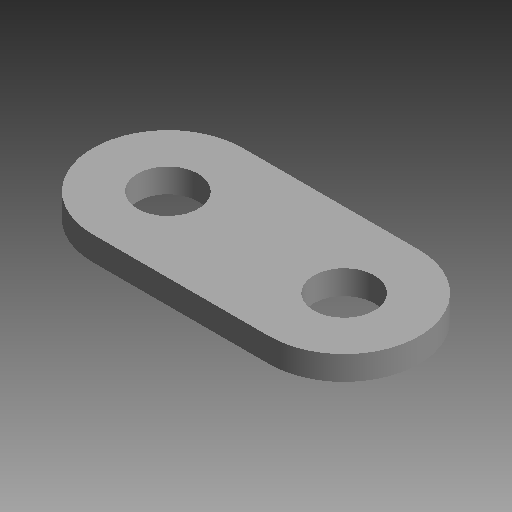
# Autodesk Inventor part: 06B - 1 RP- Link Plate
Saved by Autodesk Inventor 2019 (Build 230136000, 136)
## iProperties
Category: PARTsolutions
Company: KANA
Part Number: 06B - 1 RP- Link Plate
Material: 一般
Catalog Web Link: www.cadenas.de
Description: Standard Chain_Body1a-
Vendor: KANA
Document SubType Name: Modeling
Designer: partserver
Manufacturer: KANA
Mass: 0.145318 g
Surface Area: 3.08204 cm^2
Volume: 0.145318 cm^3
Density: 1 g/cm^3
Appearance: PSOLRGB-192-192-192
PSOL_IDENT_0: {$CADENAS_DATA\23d-libs\kana\roller_chain\standard_chain\standard_chain_body1_a.prj},194 {VTYP=3D},{
PSOL_IDENT_1: NB=06B - 1 RP- Link Plate},{LINA=06B - 1 RP},{NN=Standard Chain_Body1a},{DATE=04.07.2018 01:10:23},{
PSOL_IDENT_2: GEOMDATE=05.10.2016 10:14:00},{VERSION=},{LINEID=250},{WBVAR=NOL},{WBNUMERIC=NOL}  {NB=06B - 1 RP- L
PSOL_IDENT_3: ink Plate},{LINA=06B - 1 RP},{KT=DUMMY},{CNO=06B},{PT=RP},{NOL=1},{NOLX=1},{P=9.525},{R=6.350},{W=5.
PSOL_IDENT_4: 720},{T=1.300},{H=8.100},{D=3.280},{L=13.6},{C=10.24},{H2=8.100}
NB: 06B - 1 RP- Link Plate
NN: Standard Chain_Body1a
NBSYN: $CNO. - $NOL. $PT.- Link Plate
LINA: 06B - 1 RP
CATALOG: KANA
CNO: 06B
PT: RP
NOL: 1
P: 9.525
R: 6.35
W: 5.72
T: 1.3
H: 8.1
D: 3.28
H2: 8.1
SUPPLIER: KANA
ARTICLENO: 06B - 1 RP- Link Plate
BOMINFO: 06B - 1 RP
CREATOR: CADENAS GmbH
Title: 06B - 1 RP
Author: Cadenas PARTsolutions
Autodesk Inventor part; units mm, degrees
sketch "Sketch_4" plane through (0, 0, 0) normal (0, 0, 1) x (1, 0, 0)
  arc A0 (0, 4.05) -> (0, -4.05) centre (0, 0) ccw
  line L0 (0, -4.05) -> (9.525, -4.05)
  arc A1 (9.525, -4.05) -> (9.525, 4.05) centre (9.525, 0) ccw
  line L1 (9.525, 4.05) -> (0, 4.05)
  circle A2 centre (9.525, 0) radius 1.64
  circle A3 centre (0, 0) radius 1.64
  constraints: 4 centre point, 4 end point, 4 point on circle
extrude "Extrusion1" add sketch "Sketch_4" along normal blind 1.3
ref_plane "link_plate_XY" through (0, 0, -4.16) normal (0, 0, 1) x (1, 0, 0)
ref_plane "link_plate_YZ" through (0, 0, -4.16) normal (1, 0, 0) x (0, 1, 0)
ref_plane "link_plate_ZX" through (0, 0, -4.16) normal (0, 1, 0) x (0, 0, 1)
ref_plane "link_plate_b_XY" through (9.525, 0, -4.16) normal (0, 0, 1) x (1, 0, 0)
ref_plane "link_plate_b_YZ" through (9.525, 0, -4.16) normal (1, 0, 0) x (0, 1, 0)
ref_plane "link_plate_b_ZX" through (9.525, 0, -4.16) normal (0, 1, 0) x (0, 0, 1)
body "Solid1"
